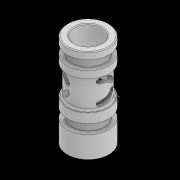
# Autodesk Inventor part: outer_sleeve
Saved by Autodesk Inventor 2021 (Build 250183000, 183)
## iProperties
Created: 2024-02-18
Part Number: outer_sleeve
Material: Generic
Document SubType Name: Modeling
Designer: top10
Density: 1 g/cm^3
Appearance: Default
Mass: 0.903098 g
Surface Area: 15.2492 cm^2
Volume: 0.903098 cm^3
Author: top10
Autodesk Inventor part; units mm, degrees
ref_plane "XZ Plane" through (0, 0, 0) normal (0, 1, 0) x (-1, 0, 0)
ref_plane "XY Plane" through (0, 0, 0) normal (0, 0, 1) x (1, 0, 0)
sketch "Sketch2" plane through (0, 0, 0) normal (0, 0, 1) x (1, 0, 0)
  line L0 (0, 7.5575) -> (0, -7.5575)
  line L1 (4, 0) -> (6, 0)
  line L2 (6, -18) -> (4.8, -18)
  line L3 (4.8, -18) -> (4.8, -20.7)
  line L4 (6, -23) -> (4, -23)
  line L5 (4.8, -20.7) -> (6, -20.7)
  line L6 (6, -20.7) -> (6, -23)
  line L7 (4, 0) -> (4, -23)
  line L8 (-7.3896, -11) -> (19.3896, -11)
  line L9 (4.375, 0) -> (5.625, 0)
  line L10 (6, 0) -> (6, -2)
  line L11 (6, -2) -> (4.8, -2)
  line L12 (4.8, -2) -> (4.8, -4.7)
  line L13 (4.8, -4.7) -> (6, -4.7)
  line L14 (6, -4.7) -> (6, -18)
  point P0 (0, 0)
  point P1 (0, 0)
  point P2 (4.75, -18)
  point P3 (6, -11)
  point P4 (6, -11)
  point P5 (5, 0)
  dimension "d2" = 23
  dimension "d64" = 8
  dimension "d74" = 11
  dimension "d77" = 9.6
  dimension "d78" = 2.7
  dimension "d84" = 12
  dimension "d86" = 2
  dimension "d90" = 18
  constraints: 31 end point, 5 midpoint, 5 perpendicular, 4 horizontal, 4 vertical, 3 vertical alignment, 2 point on line, 1 coincident, 1 collinear, 1 horizontal alignment
  measures "d2" distance between parallel lines of L4 L1
  measures "d64" diameter of L7 L0
  measures "d74" vertical distance of point (0, 0) L8.start
  measures "d77" diameter of L3 L0
  measures "d78" distance between parallel lines of L2 L5
  measures "d84" diameter of L10 L0
  measures "d86" distance of L1.end L10.end
  measures "d90" distance of L1.end L2.start
revolve "Revolution1" add sketch "Sketch2" angle 360 about axis through (0, 7.5575, 0) along (0, -1, 0)
ref_plane "Work Plane1" through (6, -11, 0) normal (1, 0, 0) x (0, 1, 0)
sketch "Sketch3" plane through (6, -11, 0) normal (1, 0, 0) x (0, 1, 0)
  line L0 (2.6181, -1.8794) -> (1.25, 1.8794) construction
  line L1 (3.5578, -1.5374) -> (2.1897, 2.2214)
  line L2 (0.3103, 1.5374) -> (1.6784, -2.2214)
  arc A0 (1.6784, -2.2214) -> (3.5578, -1.5374) centre (2.6181, -1.8794) ccw
  arc A1 (2.1897, 2.2214) -> (0.3103, 1.5374) centre (1.25, 1.8794) ccw
  line L3 (-1.25, 1.8794) -> (-2.6181, -1.8794) construction
  line L4 (-2.1897, 2.2214) -> (-3.5578, -1.5374)
  line L5 (-1.6784, -2.2214) -> (-0.3103, 1.5374)
  arc A2 (-0.3103, 1.5374) -> (-2.1897, 2.2214) centre (-1.25, 1.8794) ccw
  arc A3 (-3.5578, -1.5374) -> (-1.6784, -2.2214) centre (-2.6181, -1.8794) ccw
  line L6 (0, 4.9735) -> (0, -4.9735)
  line L7 (1.934, 0) -> (-1.934, 0)
  point P0 (11, 0)
  point P1 (0, 0)
  point P2 (0, 0)
  dimension "d13" = 2
  dimension "d14" = 2
  dimension "d15" = 20
  dimension "d16" = 20
  dimension "d18" = 4
  dimension "d32" = 2.5
  constraints: 20 end point, 8 point on circle, 8 tangent, 4 centre point, 4 horizontal alignment, 4 midpoint, 2 parallel, 1 coincident, 1 horizontal, 1 vertical
  measures "d13" distance between parallel lines of L1 L2
  measures "d14" distance between parallel lines of L5 L4
  measures "d15" angle of L6 L0
  measures "d16" angle of L6 L3
  measures "d18" distance of L0.end L0.start
  measures "d32" distance of L3.start L0.end
extrude "Extrusion1" [suppressed]
sketch "Sketch4" plane through (0, 0, 0) normal (0, 0, 1) x (1, 0, 0)
  line L0 (6, -6.75) -> (5.25, -6.75)
  line L1 (5.25, -6.75) -> (5.25, -15.25)
  line L2 (5.25, -15.25) -> (6, -15.25)
  line L3 (6, -15.25) -> (6, -6.75)
  line L4 (0, 4.6) -> (0, -27.6) projected
  line L5 (-7.3896, -11) -> (19.3896, -11) projected
  line L6 (6, -4.7) -> (6, -18) projected
  point P0 (0, 0)
  point P1 (5.25, -11)
  dimension "d75" = 8.5
  dimension "d80" = 0.75
  constraints: 8 end point, 2 parallel, 2 point on line, 1 horizontal, 1 midpoint, 1 perpendicular
  measures "d75" distance between parallel lines of L0 L2
  measures "d80" distance between parallel lines of L3 L1
revolve "Revolution2" cut sketch "Sketch4" angle 360 about axis through (0, -11.5, 0) along (0, -1, 0)
fillet "Fillet1" radius 0.5 2 edges at (-5.25, -6.75, 0) (-5.25, -15.25, 0)
pattern_circular "Circular Pattern1" [suppressed]
ref_plane "Work Plane3" through (0, 7.5575, 0) normal (0, 0, 1) x (0, -1, 0)
sketch "Sketch5" plane through (0, 7.5575, 0) normal (0, 0, 1) x (0, -1, 0)
  line L0 (0.4399, -0.05) -> (30.5575, -0.05)
  line L1 (30.5575, -0.05) -> (30.5575, 0.05)
  line L2 (30.5575, 0.05) -> (0.4399, 0.05)
  line L3 (0.4399, 0.05) -> (0.4399, -0.05)
  line L4 (0, 0) -> (15.1149, 0) projected
  line L5 (30.5575, -4) -> (30.5575, 4) projected
  point P0 (7.5575, 0)
  point P1 (30.5575, 0)
  dimension "d34" = 0.1
  constraints: 8 end point, 2 parallel, 1 horizontal, 1 horizontal alignment, 1 midpoint, 1 perpendicular, 1 point on line
  measures "d34" distance between parallel lines of L0 L2
extrude "Extrusion2" [suppressed]
feature "Unwrap1" [suppressed]
chamfer "Chamfer3" distance 0.25 angle 45 2 edges at (-6, 0, 0) (-4, 0, 0)
sketch "Sketch10" plane through (0, -23, 0) normal (0, -1, 0) x (1, 0, 0)
  circle A0 centre (0, 0) radius 4.5
  circle A1 centre (0, 0) radius 6 projected
  point P0 (0, 0)
  dimension "d59" = 9
  constraints: 1 centre point, 1 coincident
  measures "d59" diameter of A0
extrude "Extrusion6" add sketch "Sketch10" along normal blind 4
chamfer "Chamfer5" distance 0.5 angle 45 1 edges at (-4.5, -27, 0)
chamfer "Chamfer6" distance 0.2 angle 45 1 edges at (-4, -23, 0)
ref_plane "Work Plane4" through (6, -11, 0) normal (1, 0, 0) x (0, 1, 0)
sketch "Sketch13" plane through (6, -11, 0) normal (1, 0, 0) x (0, 1, 0)
  spline S0 degree 3 poles (-2.0587, 1.599) (-2.1007, 1.008) (-2.0036, 0.4034) (-1.5445, -0.6816) (-1.1887, -1.1442) (-0.7365, -1.4942) knots 0 0 0 0 0.5 0.5 1 1 1 1
  spline S1 degree 3 poles (-3.4762, 1.7383) (-3.4518, 1.9198) (-3.3581, 2.0824) (-3.213, 2.1938) (-3.0679, 2.3052) (-2.8833, 2.3569) (-2.6988, 2.3393) (-2.5143, 2.3218) (-2.3441, 2.2361) (-2.2247, 2.0986) (-2.1052, 1.9611) (-2.0459, 1.7819) (-2.0587, 1.599) knots 0 0 0 0 0.25 0.25 0.25 0.5 0.5 0.5 0.75 0.75 0.75 1 1 1 1
  spline S2 degree 3 poles (-1.636, -2.4245) (-1.7511, -2.3467) (-1.8736, -2.2619) (-2.1015, -2.0906) (-2.2097, -2.0028) (-2.3816, -1.8423) (-2.4487, -1.7731) (-2.5925, -1.6116) (-2.6706, -1.5128) (-2.8431, -1.2692) (-2.9351, -1.1185) (-3.0633, -0.8746) (-3.1064, -0.7847) (-3.2266, -0.5091) (-3.294, -0.3179) (-3.3895, 0.0292) (-3.4228, 0.1812) (-3.4876, 0.5655) (-3.5108, 0.8032) (-3.5177, 1.1566) (-3.5156, 1.2746) (-3.5055, 1.4443) (-3.5014, 1.4933) (-3.4907, 1.6066) (-3.4836, 1.6726) (-3.4762, 1.7383) knots 0 0 0 0 0.091299 0.091299 0.178822 0.178822 0.239108 0.239108 0.320725 0.320725 0.430895 0.430895 0.493589 0.493589 0.619605 0.619605 0.714672 0.714672 0.856279 0.856279 0.926137 0.926137 0.957552 0.957552 1 1 1 1
  spline S3 degree 3 poles (-0.7365, -1.4942) (-0.5963, -1.6034) (-0.5084, -1.754) (-0.4759, -2.0685) (-0.5324, -2.2192) (-0.7665, -2.4481) (-0.937, -2.5187) (-1.3017, -2.5513) (-1.4898, -2.5122) (-1.636, -2.4245) knots 0 0 0 0 0.25 0.25 0.5 0.5 0.75 0.75 1 1 1 1
  spline S4 degree 3 poles (0.7359, -1.4942) (1.1881, -1.1442) (1.5439, -0.6816) (2.003, 0.4033) (2.1002, 1.008) (2.0582, 1.599) knots 0 0 0 0 0.5 0.5 1 1 1 1
  spline S5 degree 3 poles (2.0582, 1.599) (2.0457, 1.7824) (2.1046, 1.9611) (2.2241, 2.0986) (2.3435, 2.2361) (2.5156, 2.3219) (2.6983, 2.3393) (2.8809, 2.3568) (3.0673, 2.3052) (3.2124, 2.1938) (3.3575, 2.0824) (3.4517, 1.9193) (3.4756, 1.7383) knots 0 0 0 0 0.25 0.25 0.25 0.5 0.5 0.5 0.75 0.75 0.75 1 1 1 1
  spline S6 degree 3 poles (3.4756, 1.7383) (3.4805, 1.6701) (3.4846, 1.61) (3.4898, 1.5323) (3.4913, 1.5085) (3.4934, 1.4758) (3.494, 1.4655) (3.4949, 1.4507) (3.4952, 1.4459) (3.4956, 1.4389) (3.4957, 1.4366) (3.496, 1.4321) (3.4961, 1.4313) (3.4996, 1.3699) (3.5022, 1.315) (3.5053, 1.2369) (3.5061, 1.2116) (3.5071, 1.1747) (3.5075, 1.1626) (3.508, 1.1387) (3.5082, 1.1293) (3.5093, 1.06) (3.5093, 1.0062) (3.5077, 0.9022) (3.5061, 0.8546) (3.5007, 0.7524) (3.497, 0.701) (3.4873, 0.5973) (3.4811, 0.5427) (3.4611, 0.3923) (3.444, 0.2911) (3.402, 0.0875) (3.3764, -0.0176) (3.2925, -0.3188) (3.2252, -0.5103) (2.9856, -1.0628) (2.7776, -1.3942) (2.4546, -1.7636) (2.3879, -1.834) (2.2503, -1.9682) (2.1809, -2.0307) (2.0692, -2.1234) (2.0315, -2.1533) (1.9742, -2.197) (1.955, -2.2113) (1.926, -2.2324) (1.9163, -2.2394) (1.9018, -2.2498) (1.8969, -2.2533) (1.8872, -2.2602) (1.8808, -2.2647) (1.8235, -2.3047) (1.7428, -2.3577) (1.6354, -2.4245) knots 0 0 0 0 0.03125 0.03125 0.046875 0.046875 0.054688 0.054688 0.058594 0.058594 0.060547 0.060547 0.0625 0.0625 0.09375 0.09375 0.109375 0.109375 0.117188 0.117188 0.125 0.125 0.15625 0.15625 0.1875 0.1875 0.21875 0.21875 0.25 0.25 0.3125 0.3125 0.375 0.375 0.5 0.5 0.75 0.75 0.8125 0.8125 0.875 0.875 0.90625 0.90625 0.921875 0.921875 0.929688 0.929688 0.933594 0.933594 0.9375 0.9375 1 1 1 1
  spline S7 degree 3 poles (1.6354, -2.4245) (1.4877, -2.5126) (1.303, -2.5514) (1.1188, -2.535) (0.9347, -2.5185) (0.766, -2.4481) (0.6489, -2.3337) (0.5318, -2.2192) (0.4754, -2.0685) (0.4916, -1.9112) (0.5078, -1.754) (0.5958, -1.6028) (0.7359, -1.4942) knots 0 0 0 0 0.25 0.25 0.25 0.5 0.5 0.5 0.75 0.75 0.75 1 1 1 1
  line L0 (-3.3796, 0) -> (3.3796, 0) construction
  point P0 (11, 0)
  point P1 (2.0563, -6.8828)
  point P2 (0, 0)
  point P3 (0, 0)
  constraints: 2 end point, 1 midpoint, 18 other
extrude "Extrusion8" cut sketch "Sketch13" against normal up to surface round surface about axis through (0, -11.5, 0) along (0, -1, 0) radius 4 far side no
pattern_circular "Circular Pattern3" count 3 over 360 about axis through (0, -11.5, 0) along (0, -1, 0) of "Extrusion8"
equation "\"d14\" = d13"
equation "\"d16\" = d15"
body "Solid1"
body "Srf1"
